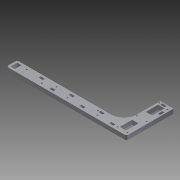
# Autodesk Inventor part: brazo eje z
Saved by Autodesk Inventor 2012 SP1 (Build 160190100, 190)
## iProperties
Created: 2014-12-27
Part Number: brazo eje z
Material: Default
Document SubType Name: Modeling
Designer: PRINCIPAL
Density: 1 g/cm^3
Author: PRINCIPAL
Autodesk Inventor part; units mm, degrees
ref_plane "YZ Plane" through (0, 0, 0) normal (1, 0, 0) x (0, 1, 0)
ref_plane "XZ Plane" through (0, 0, 0) normal (0, 1, 0) x (-1, 0, 0)
ref_plane "XY Plane" through (0, 0, 0) normal (0, 0, 1) x (1, 0, 0)
sketch "Boceto1" plane through (0, 0, 0) normal (0, 0, 1) x (1, 0, 0)
  line L0 (0, 0) -> (220, 0)
  line L1 (251, 0) -> (251, -25)
  line L2 (251, -25) -> (0, -25)
  line L3 (220, 0) -> (220, 85)
  line L4 (220, 85) -> (251, 85)
  line L5 (251, 85) -> (251, 0)
  line L6 (0, -25) -> (-30, -25)
  line L7 (-30, -25) -> (-30, 0)
  line L8 (-30, 0) -> (0, 0)
  dimension "d3" = 85
  dimension "d4" = 31
  constraints: 18 end point, 3 parallel, 3 perpendicular, 1 horizontal
  measures "d3" distance between parallel lines of L4 L0
  measures "d4" distance between parallel lines of L5 L3
extrude "Extrusión1" add sketch "Boceto1" along normal blind 10
fillet "Empalme1" radius 30 1 edges at (220, 0, 5)
sketch "Boceto2" plane through (0, 0, 10) normal (0, 0, 1) x (1, 0, 0)
  line L0 (220, 30) -> (220, 85) projected
  line L1 (251, -25) -> (-30, -25) projected
  line L2 (220, 85) -> (251, 85) projected
  line L3 (225.1, 75) -> (239.9, 75)
  line L4 (239.9, 75) -> (239.9, 46)
  line L5 (239.9, 46) -> (225.1, 46)
  line L6 (225.1, 46) -> (225.1, 75)
  line L7 (225.1, 14) -> (239.9, 14)
  line L8 (239.9, 14) -> (239.9, -15)
  line L9 (239.9, -15) -> (225.1, -15)
  line L10 (225.1, -15) -> (225.1, 14)
  point P0 (225, 80)
  point P1 (220, 75)
  point P2 (5, -25)
  point P3 (240, -25)
  point P4 (245, -20)
  point P5 (245, 75)
  point P6 (240, 80)
  point P7 (0, 0)
  point P8 (0, -25)
  dimension "d10" = 14.8
  dimension "d11" = 14.8
  dimension "d12" = 5.1
  dimension "d14" = 10
  dimension "d15" = 29
  dimension "d16" = 29
  dimension "d17" = 10
  dimension "d82" = 5.1
  constraints: 16 end point, 4 parallel, 2 horizontal, 2 perpendicular, 1 other
  measures "d10" distance between parallel lines of L8 L10
  measures "d11" distance between parallel lines of L4 L6
  measures "d12" distance between parallel lines of L6 L0
  measures "d15" distance between parallel lines of L5 L3
  measures "d16" distance between parallel lines of L9 L7
  measures "d17" distance between parallel lines of L1 L9
  measures "d82" distance between parallel lines of L10 L0
extrude "Extrusión2" cut sketch "Boceto2" against normal blind 10
sketch "Boceto3" plane through (0, 0, 10) normal (0, 0, 1) x (1, 0, 0)
  line L0 (0, 0) -> (190, 0) projected
  line L1 (251, -25) -> (-30, -25) projected
  line L2 (180, -10) -> (170, -10)
  line L3 (170, -10) -> (170, -5)
  line L4 (170, -5) -> (180, -5)
  line L5 (180, -5) -> (180, -10)
  line L6 (110, -5) -> (100, -5)
  line L7 (100, -5) -> (100, -10)
  line L8 (100, -10) -> (110, -10)
  line L9 (110, -10) -> (110, -5)
  line L10 (40, -5) -> (30, -5)
  line L11 (30, -5) -> (30, -10)
  line L12 (30, -10) -> (40, -10)
  line L13 (40, -10) -> (40, -5)
  line L14 (145, -15) -> (135, -15)
  line L15 (135, -15) -> (135, -20)
  line L16 (135, -20) -> (145, -20)
  line L17 (145, -20) -> (145, -15)
  line L18 (75, -15) -> (65, -15)
  line L19 (65, -15) -> (65, -20)
  line L20 (65, -20) -> (75, -20)
  line L21 (75, -20) -> (75, -15)
  point P0 (5, 0)
  point P1 (0, -5)
  point P2 (0, -20)
  point P3 (5, -25)
  point P4 (240, -25)
  dimension "d20" = 10
  dimension "d21" = 10
  dimension "d22" = 10
  dimension "d24" = 5
  dimension "d25" = 5
  dimension "d26" = 5
  dimension "d27" = 5
  dimension "d28" = 5
  dimension "d29" = 10
  dimension "d30" = 10
  dimension "d31" = 5
  dimension "d32" = 5
  dimension "d33" = 5
  dimension "d34" = 5
  dimension "d36" = 25
  dimension "d37" = 25
  dimension "d38" = 25
  dimension "d39" = 25
  constraints: 40 end point, 10 parallel, 5 horizontal, 5 perpendicular
  measures "d20" distance between parallel lines of L13 L11
  measures "d21" distance between parallel lines of L9 L7
  measures "d22" distance between parallel lines of L5 L3
  measures "d24" distance between parallel lines of L0 L6
  measures "d25" distance between parallel lines of L0 L4
  measures "d26" distance between parallel lines of L4 L2
  measures "d27" distance between parallel lines of L6 L8
  measures "d28" distance between parallel lines of L10 L12
  measures "d29" distance between parallel lines of L21 L19
  measures "d30" distance between parallel lines of L17 L15
  measures "d31" distance between parallel lines of L14 L16
  measures "d32" distance between parallel lines of L1 L16
  measures "d33" distance between parallel lines of L1 L20
  measures "d34" distance between parallel lines of L20 L18
  measures "d36" distance between parallel lines of L19 L13
  measures "d37" distance between parallel lines of L21 L7
  measures "d38" distance between parallel lines of L9 L15
  measures "d39" distance between parallel lines of L3 L17
extrude "Extrusión3" cut sketch "Boceto3" against normal blind 10
sketch "Boceto4" plane through (0, 0, 10) normal (0, 0, 1) x (1, 0, 0)
  line L0 (145, -15) -> (145, -20) projected
  line L1 (145, -20) -> (135, -20) projected
  line L2 (205, -20) -> (215, -20)
  line L3 (215, -20) -> (215, -15)
  line L4 (215, -15) -> (205, -15)
  line L5 (205, -15) -> (205, -20)
  point P0 (0, 0)
  dimension "d42" = 10
  dimension "d43" = 5
  dimension "d44" = 60
  constraints: 8 end point, 2 parallel, 1 horizontal, 1 perpendicular, 1 point on line
  measures "d42" distance between parallel lines of L3 L5
  measures "d43" distance between parallel lines of L2 L4
  measures "d44" distance between parallel lines of L0 L5
extrude "Extrusión4" cut sketch "Boceto4" against normal blind 10
sketch "Boceto6" plane through (0, 0, 10) normal (0, 0, 1) x (1, 0, 0)
  line L0 (237.5, 82.5) -> (227.5, 82.5)
  line L1 (227.5, 82.5) -> (227.5, 77.5)
  line L2 (227.5, 77.5) -> (237.5, 77.5)
  line L3 (237.5, 77.5) -> (237.5, 82.5)
  circle A0 centre (245.5, -17.5) radius 1.6
  circle A1 centre (245.5, 27.5) radius 1.6
  circle A2 centre (245.5, 75.9891) radius 1.6
  circle A3 centre (222.4918, 80) radius 1.6
  circle A4 centre (222.4918, 27.5) radius 1.6
  circle A5 centre (175, -17.5) radius 1.6
  circle A6 centre (166.25, -7.5) radius 1.6
  circle A7 centre (105, -17.5) radius 1.6
  circle A8 centre (70, -7.5) radius 1.6
  circle A9 centre (45, -17.5) radius 1.6
  circle A10 centre (0, -7.5) radius 1.6
  line L4 (-30, -25) -> (-30, 0) projected
  circle A11 centre (222.4918, -17.5) radius 1.6
  line L5 (251, 85) -> (251, -25) projected
  line L6 (220, 85) -> (251, 85) projected
  line L7 (170, -10) -> (170, -5) projected
  point P0 (0, 0)
  dimension "d52" = 5
  dimension "d54" = 3.2
  dimension "d55" = 3.2
  dimension "d56" = 3.2
  dimension "d57" = 3.2
  dimension "d58" = 3.2
  dimension "d60" = 3.2
  dimension "d61" = 3.2
  dimension "d62" = 3.2
  dimension "d63" = 3.2
  dimension "d64" = 3.2
  dimension "d65" = 3.2
  dimension "d80" = 30
  dimension "d81" = 3.2
  dimension "d83" = 5.5
  dimension "d84" = 5.5
  dimension "d85" = 5.5
  dimension "d92" = 2.5
  dimension "d93" = 5
  dimension "d94" = 3.75
  dimension "d95" = 75
  constraints: 12 centre point, 8 end point, 2 parallel, 1 horizontal, 1 perpendicular
  measures "d52" distance between parallel lines of L0 L2
  measures "d54" diameter of A0
  measures "d55" diameter of A1
  measures "d56" diameter of A2
  measures "d57" diameter of A3
  measures "d58" diameter of A4
  measures "d60" diameter of A5
  measures "d61" diameter of A6
  measures "d62" diameter of A7
  measures "d63" diameter of A8
  measures "d64" diameter of A9
  measures "d65" diameter of A10
  measures "d80" distance from line of A10.centre L4
  measures "d81" diameter of A11
  measures "d83" distance from line of A0.centre L5
  measures "d84" distance from line of L5 A1.centre
  measures "d85" distance from line of L5 A2.centre
  measures "d92" distance between parallel lines of L0 L6
  measures "d93" distance from line of L6 A3.centre
  measures "d94" distance from line of A6.centre L7
  measures "d95" distance from line of A9.centre L4
extrude "Extrusión6" cut sketch "Boceto6" against normal blind 10
fillet "Empalme3" radius 5 1 edges at (251, -25, 5)
fillet "Empalme4" radius 5 2 edges at (-30, 0, 5) (-30, -25, 5)
fillet "Empalme5" radius 1 2 edges at (220, 85, 5) (251, 85, 5)
sketch "Boceto7" plane through (0, 0, 10) normal (0, 0, 1) x (1, 0, 0)
  line L0 (-25, 0) -> (190, 0) projected
  line L1 (-30, -20) -> (-30, -5) projected
  line L2 (-25, -5) -> (-15, -5)
  line L3 (-15, -5) -> (-15, -20)
  line L4 (-15, -20) -> (-25, -20)
  line L5 (-25, -20) -> (-25, -5)
  point P0 (0, 0)
  dimension "d74" = 10
  dimension "d75" = 15
  dimension "d76" = 5
  dimension "d77" = 5
  constraints: 8 end point, 2 parallel, 1 horizontal, 1 perpendicular
  measures "d74" distance of L3.end L4.end
  measures "d75" distance between parallel lines of L4 L2
  measures "d76" distance between parallel lines of L0 L2
  measures "d77" distance between parallel lines of L1 L5
extrude "Extrusión7" cut sketch "Boceto7" against normal blind 10
sketch "Boceto8" plane through (0, 0, 10) normal (0, 0, 1) x (1, 0, 0)
  line L0 (221, 85) -> (250, 85) projected
  line L1 (251, 84) -> (251, -20) projected
  line L2 (243, 66.5) -> (248, 66.5)
  line L3 (248, 66.5) -> (248, 56.5)
  line L4 (248, 56.5) -> (243, 56.5)
  line L5 (243, 56.5) -> (243, 66.5)
  point P0 (0, 0)
  dimension "d86" = 5
  dimension "d87" = 10
  dimension "d88" = 3
  dimension "d89" = 18.5
  constraints: 8 end point, 2 parallel, 1 horizontal, 1 perpendicular
  measures "d86" distance of L3.end L4.end
  measures "d87" distance of L2.end L3.end
  measures "d88" distance between parallel lines of L3 L1
  measures "d89" distance between parallel lines of L0 L2
extrude "Extrusión8" cut sketch "Boceto8" against normal blind 10
